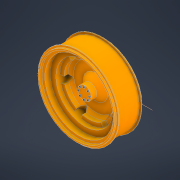
# Autodesk Inventor part: McCrea_koleso_jadro_walle
Saved by Autodesk Inventor 2022 (Build 260153000, 153)
## iProperties
Created: 2022-02-21
Part Number: McCrea_koleso_jadro_walle
Material: Generic
Document SubType Name: Modeling
Designer: MatusBarany
Density: 1 g/cm^3
Appearance: Default
Author: MatusBarany
Autodesk Inventor part; units mm, degrees
ref_plane "YZ Plane" through (0, 0, 0) normal (1, 0, 0) x (0, 1, 0)
sketch "Sketch1" plane through (0, 0, 0) normal (0, 0, 1) x (1, 0, 0)
  circle A0 centre (0, 0) radius 140
  dimension "d0" = 280
  constraints: 1 centre point, 1 coincident
  measures "d0" diameter of A0
extrude "Extrusion1" add sketch "Sketch1" along normal blind 30
sketch "Sketch2" plane through (0, 0, 30) normal (0, 0, 1) x (1, 0, 0)
  circle A0 centre (0, 0) radius 140 projected
  circle A1 centre (0, 0) radius 125
  dimension "d3" = 15
  constraints: 1 centre point, 1 coincident
  measures "d3" radial gap between concentric circles of A0 A1
extrude "Extrusion2" add sketch "Sketch2" along normal blind 60
sketch "Sketch3" plane through (0, 0, 90) normal (0, 0, 1) x (1, 0, 0)
  circle A0 centre (0, 0) radius 125 projected
  circle A1 centre (0, 0) radius 135
  circle A2 centre (0, 0) radius 140 projected
  dimension "d6" = 5
  constraints: 1 centre point, 1 coincident
  measures "d6" radial gap between concentric circles of A2 A1
extrude "Extrusion3" add sketch "Sketch3" along normal blind 10 contours A2
sketch "Sketch4" plane through (0, 0, 30) normal (0, 0, 1) x (1, 0, 0)
  circle A0 centre (0, 0) radius 125 projected
  circle A1 centre (0, 0) radius 105
  circle A2 centre (0, 0) radius 25
  dimension "d9" = 20
  dimension "d10" = 50
  constraints: 2 centre point, 2 coincident
  measures "d9" radial gap between concentric circles of A0 A1
  measures "d10" diameter of A2
extrude "Extrusion4" add sketch "Sketch4" along normal blind 40
sketch "Sketch5" plane through (0, 0, 30) normal (0, 0, 1) x (1, 0, 0)
  arc A0 (-63.63961, 63.63961) -> (-90, 0) centre (0, 0) ccw
  line L0 (-90, 0) -> (-105, 0)
  circle A1 centre (0, 0) radius 105
  line L1 (-196, 0) -> (196, 0)
  line L2 (-63.63961, 63.63961) -> (-74.246212, 74.246212)
  dimension "d13" = 90
  dimension "d14" = 45
  dimension "d16" = 45
  constraints: 4 end point, 4 point on circle, 1 centre point, 1 coincident, 1 collinear
  measures "d13" radius of A0
  measures "d16" angle of L2 L0
extrude "Extrusion5" add sketch "Sketch5" along normal blind 25 contours A0 L0 A1 L2
pattern_circular "Circular Pattern1" count 6 over 360 about axis through (0, 0, 30) along (0, 0, 1) of "Extrusion5"
chamfer "Chamfer1" distance 20 angle 45 1 edges at (-25, 0, 30)
chamfer "Chamfer2" distance 10 angle 45 17 edges at (-83.1492, 34.4415, 30) (25.2349, 94.1778, 30) (-11.7474, 89.23, 30) (-48.75, 84.4375, 30) (-68.9429, 68.9429, 30) (-97.5, 0, 30) (-94.1778, -25.2349, 30) (-71.4018, -54.7885, 30) (11.7474, -89.23, 30) (71.4018, 54.7885, 30) (83.1492, -34.4415, 30) (94.1778, 25.2349, 30) (97.5, 0, 30) (48.75, -84.4375, 30) (-48.75, -84.4375, 30) (48.75, 84.4375, 30) (-25.2349, -94.1778, 30)
sketch "Sketch6" plane through (0, 0, 70) normal (0, 0, 1) x (1, 0, 0)
  circle A0 centre (0, -20) radius 3.5
  circle A1 centre (0, 0) radius 25
  circle A2 centre (0, 0) radius 25
  line L0 (0, -25) -> (0, 25) construction
  circle A3 centre (14.142136, -14.142136) radius 3.5
  circle A4 centre (20, 0) radius 3.5
  circle A5 centre (14.142136, 14.142136) radius 3.5
  circle A6 centre (0, 20) radius 3.5
  circle A7 centre (-14.142136, 14.142136) radius 3.5
  circle A8 centre (-20, 0) radius 3.5
  circle A9 centre (-14.142136, -14.142136) radius 3.5
  dimension "d31" = 50
  dimension "d32" = 50
  dimension "d33" = 7
  dimension "d34" = 20
  dimension "d37" = 360
  constraints: 8 centre point, 2 end point, 2 point on circle, 1 point on line, 1 vertical, 17 other
  measures "d31" distance of L0.start L0.end
  measures "d32" diameter of A1
  measures "d33" diameter of A0
  measures "d34" distance of A1.centre A0.centre
extrude "Extrusion6" add sketch "Sketch6" along normal blind 3 contours A0 | A3 | A4 | A5 | A6 | A7 | A8 | A9
ref_plane "Work Plane2" through (0, 0, 50) normal (0, 0, -1) x (-1, 0, 0)
ref_plane "Work Plane3" through (0, 0, 10) normal (0, 0, -1) x (-1, 0, 0)
sketch "Sketch7" plane through (0, 0, 10) normal (0, 0, -1) x (-1, 0, 0)
  circle A0 centre (0, 0) radius 147
  circle A1 centre (0, 0) radius 140 projected
  dimension "d43" = 7
  constraints: 1 centre point, 1 coincident
  measures "d43" radial gap between concentric circles of A1 A0
extrude "Extrusion7" add sketch "Sketch7" along normal blind 3
mirror "Mirror1" about plane through (0, 0, 50) normal (0, 0, -1) of "Extrusion7"
equation "\"d16\" = d14"
equation "\"d31\" = d32"
body "Solid1"
